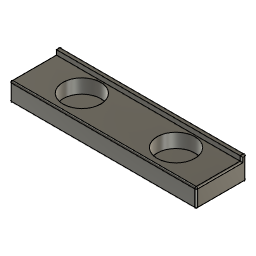
sm-vise-jaws (Autodesk Fusion 360 design; units mm, degrees)
Autodesk Fusion 360 part; units mm, degrees
box "BoxPrimitive1" add length 13.4874 width 50.292 height 5.08 placed x (0, -1, 0) y (1, 0, 0) z (0, 0, 1) at (0, 0, 0)
sketch "Sketch2" plane through (0, 0, 5.08) normal (0, 0, 1) x (-1, 0, 0)
  line L0 (0, 13.4874) -> (-50.292, 13.4874)
  line L1 (-50.292, 13.4874) -> (-50.292, 0)
  line L2 (-50.292, 0) -> (0, 0)
  line L3 (0, 0) -> (0, 13.4874)
  line L4 (-25.146, 0) -> (-25.146, 13.4874) construction
  line L5 (0, 6.7437) -> (-50.292, 6.7437) construction
  line L6 (-12.7, 0) -> (-12.7, 13.4874) construction
  line L7 (-38.1, 0) -> (-38.1, 13.4874) construction
  line L8 (0, 1.27) -> (-50.292, 1.27)
  point P0 (-12.7, 6.7437)
  point P1 (-38.1, 6.7437)
  constraint midpoint L2 L4.start
  constraint midpoint L0 L4.end
  constraint midpoint L3 L5.start
  constraint midpoint L1 L5.end
  constraint coincident L2 L6.start
  constraint coincident L0 L6.end
  constraint perpendicular L0 L6
  constraint coincident L2 L7.start
  constraint coincident L0 L7.end
  constraint perpendicular L0 L7
  constraint midpoint L6 P0
  constraint midpoint L7 P1
  constraint coincident L3 L8.start
  constraint coincident L1 L8.end
  constraint perpendicular L1 L8
hole "Hole1" at (12.7, -6.7437, 5.08) direction (0, 0, -1) diameter 10.16 depth 3.81 tip angle 180
hole "Hole2" at (38.1, -6.7437, 5.08) direction (0, 0, -1) diameter 10.16 depth 3.81 tip angle 180
extrude "Extrude1" add sketch "Sketch2" along normal blind 1.27 contours L1 L2 L3 L8
fillet "Fillet1" radius 0.381 5 faces at (50.292, -4.9191, 1.6933) (33.528, 0, 2.1167) (33.528, -4.4958, 0) (0, -4.9191, 1.6933) (16.764, -13.4874, 1.6933)
